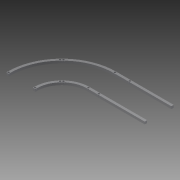
# Autodesk Inventor part: Runner Rails v2
Saved by Autodesk Inventor 2013 (Build 170138000, 138)
## iProperties
Created: 2013-01-15
Part Number: Runner Rails v2
Material: Polycarbonate, Clear
Document SubType Name: Modeling
Designer: actoennies
Mass: 228.775 g
Surface Area: 660.467 cm^2
Volume: 190.646 cm^3
Density: 1.2 g/cm^3
Author: actoennies
Autodesk Inventor part; units mm, degrees
ref_plane "YZ Plane" through (0, 0, 0) normal (1, 0, 0) x (0, 1, 0)
ref_plane "XZ Plane" through (0, 0, 0) normal (0, 1, 0) x (-1, 0, 0)
ref_plane "XY Plane" through (0, 0, 0) normal (0, 0, 1) x (1, 0, 0)
sketch "Sketch1" plane through (0, 0, 0) normal (0, 1, 0) x (-1, 0, 0)
  arc A0 (0, -273.05) -> (273.05, 0) centre (0, 0) ccw
  arc A1 (0, -285.75) -> (285.75, 0) centre (0, 0) ccw
  arc A2 (0, -146.05) -> (146.05, 0) centre (0, 0) ccw
  arc A3 (0, -133.35) -> (133.35, 0) centre (0, 0) ccw
  line L0 (0, -285.75) -> (-6.35, -285.75)
  line L1 (146.05, 0) -> (146.05, 6.35)
  line L2 (133.35, 0) -> (133.35, 6.35)
  line L3 (273.05, 6.35) -> (273.05, 0)
  line L4 (285.75, 6.35) -> (285.75, 0)
  circle A4 centre (103.1708, -94.1906) radius 3.3782
  circle A5 centre (94.1906, -103.1708) radius 3.3782
  circle A6 centre (279.4, 0) radius 3.3782
  circle A7 centre (139.7, 0) radius 3.3782
  circle A8 centre (202.0047, -193.0245) radius 3.3782
  circle A9 centre (193.0245, -202.0047) radius 3.3782
  circle A10 centre (0, -279.4) radius 3.3782
  circle A11 centre (0, -139.7) radius 3.3782
  circle A12 centre (-55.2746, -139.7) radius 3.3782
  circle A13 centre (-78.3684, -279.4) radius 3.3782
  line L5 (285.75, 6.35) -> (273.05, 6.35)
  line L6 (146.05, 6.35) -> (133.35, 6.35)
  line L7 (-314.96, -285.75) -> (-314.96, -273.05)
  line L8 (-101.6, -133.35) -> (-127, -133.35)
  line L9 (-127, -146.05) -> (-101.6, -146.05)
  line L10 (-314.96, -146.05) -> (-314.96, -133.35)
  line L11 (-6.35, -285.75) -> (-6.35, -393.7)
  line L12 (-6.35, -393.7) -> (-314.325, -393.7)
  line L13 (-314.325, -393.7) -> (-314.325, -76.2)
  line L14 (-314.325, -76.2) -> (-120.65, -76.2)
  line L15 (-120.65, -76.2) -> (0, -133.35)
  line L16 (0, -285.75) -> (-6.35, -285.75)
  line L17 (0, -146.05) -> (0, -273.05)
  dimension "d10" = 12.7
  dimension "d11" = 12.7
  dimension "d13" = 12.7
  dimension "d14" = 6.7564
  dimension "d15" = 6.7564
  dimension "d16" = 6.7564
  dimension "d18" = 6.7564
  dimension "d20" = 6.35
  dimension "d21" = 6.7564
  dimension "d22" = 6.7564
  dimension "d23" = 6.7564
  dimension "d26" = 6.7564
  dimension "d30" = 6.7564
  dimension "d32" = 6.7564
  dimension "d66" = 25.4
  dimension "d67" = 0
  dimension "d72" = 12.7
  dimension "d81" = 107.95
  dimension "d82" = 133.35
  dimension "d83" = 279.4
  dimension "d84" = 6.35
  dimension "d85" = 317.5
  dimension "d86" = 193.675
  dimension "d87" = 55.2746
  dimension "d88" = 139.7
  dimension "d91" = 307.975
  constraints: 36 end point, 14 centre point, 9 point on circle, 4 perpendicular, 3 coincident, 2 collinear, 2 parallel, 2 tangent, 1 horizontal, 1 point on line, 1 vertical, 2 other
  measures "d10" distance between parallel lines of L1 L2
  measures "d11" distance between parallel lines of L3 L4
  measures "d13" distance of L9.end L8.start
  measures "d14" diameter of A4
  measures "d15" diameter of A5
  measures "d16" diameter of A6
  measures "d18" diameter of A7
  measures "d20" distance from line of L1 A7.centre
  measures "d21" diameter of A8
  measures "d22" diameter of A9
  measures "d23" diameter of A10
  measures "d26" diameter of A11
  measures "d30" diameter of A12
  measures "d32" diameter of A13
  measures "d66" distance of L8.start L8.end
  measures "d67" vertical distance of L8.end L8.start
  measures "d72" distance of L9.start L8.end
  measures "d81" distance of L0.end L11.end
  measures "d82" horizontal distance of L2.start A10.centre
  measures "d83" distance of A0.centre A10.centre
  measures "d84" distance from line of A10.centre L11
  measures "d85" distance of L12.end L13.end
  measures "d86" distance of L13.end L14.end
  measures "d87" distance of A11.centre A12.centre
  measures "d88" vertical distance of A1.centre A12.centre
  measures "d91" distance of L11.end L12.end
extrude "Extrusion7" add sketch "Sketch1" along normal blind 6.35
sketch "Sketch7" plane through (0, 0, 0) normal (0, -1, 0) x (1, 0, 0)
  line L0 (0, -273.05) -> (0, -146.05) projected
  line L1 (314.325, -76.2) -> (314.325, -393.7) projected
  line L2 (314.325, -234.95) -> (0, -234.95)
  line L3 (301.625, -139.7) -> (301.625, -165.1)
  line L4 (301.625, -165.1) -> (98.425, -165.1)
  line L5 (98.425, -165.1) -> (98.425, -139.7)
  line L6 (98.425, -139.7) -> (301.625, -139.7)
  line L7 (301.625, -330.2) -> (301.625, -304.8)
  line L8 (301.625, -304.8) -> (98.425, -304.8)
  line L9 (98.425, -304.8) -> (98.425, -330.2)
  line L10 (98.425, -330.2) -> (301.625, -330.2)
  dimension "d92" = 25.4
  dimension "d93" = 203.2
  dimension "d94" = 12.7
  dimension "d95" = 69.85
  constraints: 18 end point, 4 symmetric about line, 3 perpendicular, 2 parallel, 1 midpoint, 1 point on line
  measures "d92" distance of L3.start L3.end
  measures "d93" distance of L3.end L4.end
  measures "d94" distance between parallel lines of L1 L3
  measures "d95" distance between parallel lines of L2 L4
extrude "Extrusion8" cut sketch "Sketch7" against normal blind 6.35
body "Solid2"
